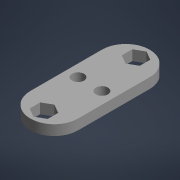
# Autodesk Inventor part: Stationary bracket aligner
Saved by Autodesk Inventor 2022 (Build 260153000, 153)
## iProperties
Created: 2022-01-30
Part Number: Stationary bracket aligner
Material: Generic
Document SubType Name: Modeling
Designer: izack
Density: 1 g/cm^3
Appearance: Default
Author: izack
## iProperties of the stored document Stationary bracket aligner_3DPrint.ipt
Part Number: Stationary bracket aligner_3DPrint
Material: Generic
Document SubType Name: Modeling
Designer: izack
Appearance: Default
Author: izack
Autodesk Inventor part; units mm, degrees
ref_plane "YZ Plane" through (0, 0, 0) normal (1, 0, 0) x (0, 1, 0)
ref_plane "XZ Plane" through (0, 0, 0) normal (0, 1, 0) x (-1, 0, 0)
ref_plane "XY Plane" through (0, 0, 0) normal (0, 0, 1) x (1, 0, 0)
sketch "Sketch1" plane through (0, 0, 0) normal (0, 1, 0) x (-1, 0, 0)
  line L0 (0, 0) -> (14, 0)
  line L1 (14, 0) -> (14, -21)
  line L2 (14, -21) -> (0, -21)
  line L3 (0, -21) -> (0, 0)
  circle A0 centre (7, 3) radius 2.65
  circle A1 centre (7, -24) radius 2.65
  circle A2 centre (7, 0) radius 7
  circle A3 centre (7, -21) radius 7
  line L4 (9.65, 1.47) -> (7, -0.06)
  line L5 (7, -0.06) -> (4.35, 1.47)
  line L6 (4.35, 1.47) -> (4.35, 4.53)
  line L7 (4.35, 4.53) -> (7, 6.06)
  line L8 (7, 6.06) -> (9.65, 4.53)
  line L9 (9.65, 4.53) -> (9.65, 1.47)
  line L10 (9.65, -25.53) -> (7, -27.06)
  line L11 (7, -27.06) -> (4.35, -25.53)
  line L12 (4.35, -25.53) -> (4.35, -22.47)
  line L13 (4.35, -22.47) -> (7, -20.94)
  line L14 (7, -20.94) -> (9.65, -22.47)
  line L15 (9.65, -22.47) -> (9.65, -25.53)
  line L16 (14, -10.5) -> (0, -10.5) construction
  circle A4 centre (10.5, -10.5) radius 1.75
  circle A5 centre (3.5, -10.5) radius 1.75
  point P0 (9.65, 3)
  point P1 (9.65, -24)
  dimension "d2" = 5.3
  dimension "d3" = 5.3
  dimension "d0" = 14
  dimension "d1" = 21
  dimension "d4" = 3
  dimension "d5" = 3
  dimension "d6" = 3.5
  dimension "d7" = 3.5
  dimension "d8" = 3.5
  dimension "d9" = 3.5
  constraints: 34 end point, 6 midpoint, 3 point on line, 2 centre point, 2 coincident, 2 horizontal alignment, 2 parallel, 1 horizontal, 1 perpendicular, 36 other
  measures "d0" distance of L1.end L2.end
  measures "d1" distance of L0.end L1.end
  measures "d4" distance from line of L2 point (7, -24)
  measures "d5" distance from line of L0 point (7, 3)
  measures "d6" diameter of A4
  measures "d7" diameter of A5
  measures "d8" distance from line of L3 A5.centre
  measures "d9" distance from line of L1 A4.centre
extrude "Extrusion1" add sketch "Sketch1" along normal blind 3 contours A2 L0 L4 L9 L8 L7 L6 L5 | A2 L1 A3 L3 | L0 L5 L4 A2 | A3 L2 L14 L13 | L2 L13 L12 L11 L10 L15 L14 A3
body "Solid1"
